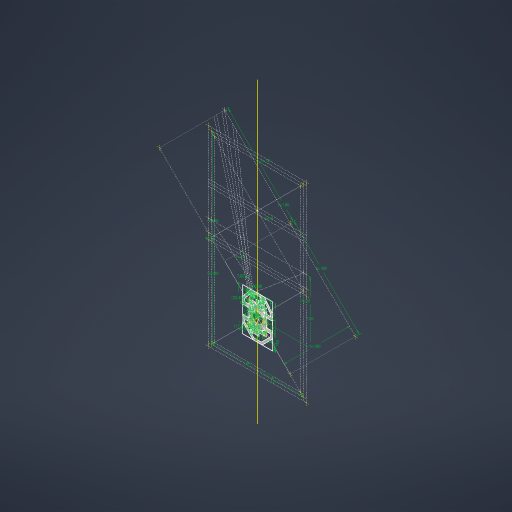
# Autodesk Inventor part: chassis
Saved by Autodesk Inventor 2023.5 (Build 275446000, 446)
## iProperties
Created: 2025-01-19
Part Number: chassis
Material: 一般
Document SubType Name: Modeling
Designer: IshiiLabHonda
Density: 1 g/cm^3
Appearance: 既定
Author: IshiiLabHonda
Autodesk Inventor part; units mm, degrees
ref_plane "YZ Plane" through (0, 0, 0) normal (1, 0, 0) x (0, 1, 0)
ref_plane "XZ Plane" through (0, 0, 0) normal (0, 1, 0) x (-1, 0, 0)
ref_plane "XY Plane" through (0, 0, 0) normal (0, 0, 1) x (1, 0, 0)
sketch "スケッチ1" plane through (0, 0, 0) normal (0, 0, 1) x (1, 0, 0)
  line L0 (-90, 90) -> (90, 90) construction
  line L1 (90, 90) -> (90, -90) construction
  line L2 (90, -90) -> (-90, -90) construction
  line L3 (-90, -90) -> (-90, 90) construction
  line L4 (-90, 90) -> (-90, 270) construction
  line L5 (-90, 270) -> (90, 270) construction
  line L6 (90, 270) -> (90, 90) construction
  line L7 (-90, 90) -> (90, -90) construction
  line L8 (90, 90) -> (-90, -90) construction
  line L9 (0, 0) -> (0, 10) construction
  line L10 (0, 0) -> (10, 0) construction
  line L11 (-90, 270) -> (90, 90) construction
  line L12 (-90, 90) -> (90, 270) construction
  line L13 (-96, 276) -> (96, 276) construction
  line L14 (96, 276) -> (96, -96) construction
  line L15 (96, -96) -> (-96, -96) construction
  line L16 (-96, -96) -> (-96, 276) construction
  line L17 (-84, 264) -> (84, 264) construction
  line L18 (84, 264) -> (84, -84) construction
  line L19 (84, -84) -> (-84, -84) construction
  line L20 (-84, -84) -> (-84, 264) construction
  line L21 (-96, 96) -> (96, 96) construction
  line L22 (-96, 84) -> (96, 84) construction
  line L23 (-63.6396, 63.6396) -> (63.6396, 190.9188) construction
  line L24 (63.6396, 190.9188) -> (190.9188, 63.6396) construction
  line L25 (190.9188, 63.6396) -> (63.6396, -63.6396) construction
  line L26 (63.6396, -63.6396) -> (-63.6396, 63.6396) construction
  line L27 (-190.9188, 190.9188) -> (-63.6396, 318.1981) construction
  line L28 (-63.6396, 318.1981) -> (63.6396, 190.9188) construction
  line L29 (-63.6396, 63.6396) -> (-190.9188, 190.9188) construction
  line L30 (-96, 120) -> (96, 120) construction
  line L31 (-96, 186) -> (96, 186) construction
  line L32 (-96, 174) -> (96, 174) construction
  line L33 (-96, 180) -> (96, 180) construction
  point P0 (-63.6396, 318.1981)
  point P1 (-90, 120)
  point P2 (90, 120)
  point P3 (0, 180)
  dimension "d8" = 10
  dimension "d9" = 10
  dimension "d10" = 12
  dimension "d11" = 12
  dimension "d12" = 12
  dimension "d13" = 12
  dimension "d14" = 180
  dimension "d15" = 180
  dimension "d16" = 180
  dimension "d17" = 12
  dimension "d34" = 180
  dimension "d35" = 180
  dimension "d36" = 180
  dimension "d37" = 120
  dimension "d85" = 12
  constraints: 68 end point, 16 parallel, 16 point on line, 9 perpendicular, 4 midpoint, 3 coincident, 1 horizontal, 7 other
  measures "d8" distance of L9.start L9.end
  measures "d9" distance of L9.start L10.end
  measures "d10" distance between parallel lines of L15 L19
  measures "d11" distance between parallel lines of L16 L20
  measures "d12" distance between parallel lines of L14 L18
  measures "d13" distance between parallel lines of L17 L13
  measures "d14" distance of L1.end L2.end
  measures "d15" distance of L2.end L0.start
  measures "d16" distance between parallel lines of L0 L5
  measures "d17" distance between parallel lines of L22 L21
  measures "d34" distance between parallel lines of L26 L24
  measures "d35" distance of L23.end L24.end
  measures "d36" distance between parallel lines of L23 L27
  measures "d37" distance between parallel lines of L10 L30
  measures "d85" distance between parallel lines of L32 L31
sketch "スケッチ2" plane through (0, 0, 0) normal (0, 0, 1) x (1, 0, 0)
  line L0 (63.6396, 190.9188) -> (190.9188, 63.6396) construction
  line L1 (-63.6396, 318.1981) -> (63.6396, 190.9188) construction
  line L2 (-84, 264) -> (84, 264) construction
  line L3 (-90, 270) -> (90, 270) construction
  line L4 (90, 270) -> (90, 90) construction
  line L5 (-96, 276) -> (96, 276) construction
  line L6 (-90, 90) -> (90, 270) construction
  line L7 (-90, 270) -> (90, 90) construction
  line L8 (-63.6396, 63.6396) -> (63.6396, 190.9188) construction
  line L9 (-96, 120) -> (96, 120) construction
  line L10 (-90, 90) -> (90, 90) construction
  line L11 (-96, 96) -> (96, 96) construction
  line L12 (-96, 84) -> (96, 84) construction
  line L13 (90, -90) -> (-90, -90) construction
  line L14 (0, 0) -> (0, 10) construction
  line L15 (0, 0) -> (10, 0) construction
  line L16 (190.9188, 63.6396) -> (63.6396, -63.6396) construction
  line L17 (63.6396, -63.6396) -> (-63.6396, 63.6396) construction
  line L18 (84, -84) -> (-84, -84) construction
  line L19 (96, -96) -> (-96, -96) construction
  line L20 (-90, 90) -> (-90, 270) construction
  line L21 (-63.6396, 63.6396) -> (-190.9188, 190.9188) construction
  line L22 (-190.9188, 190.9188) -> (-63.6396, 318.1981) construction
  line L23 (96, 276) -> (96, -96) construction
  line L24 (-96, -96) -> (-96, 276) construction
  line L25 (84, 264) -> (84, -84) construction
  line L26 (-84, -84) -> (-84, 264) construction
  line L27 (90, 90) -> (90, -90) construction
  line L28 (-90, 90) -> (90, -90) construction
  line L29 (90, 90) -> (-90, -90) construction
  line L30 (-90, -90) -> (-90, 90) construction
  circle A0 centre (0, 0) radius 16.5 construction
  circle A1 centre (0, 0) radius 10 construction
  line L31 (20, 11.5) -> (28.75, 11.5) construction
  line L32 (28.75, 11.5) -> (28.75, -11.5) construction
  line L33 (28.75, -11.5) -> (20, -11.5) construction
  line L34 (20, -11.5) -> (20, 11.5) construction
  line L35 (20, 11.5) -> (18, 11.5) construction
  line L36 (18, 11.5) -> (18, -11.5) construction
  line L37 (18, -11.5) -> (20, -11.5) construction
  line L38 (18, 1.5) -> (17, 1.5) construction
  line L39 (17, -1.5) -> (18, -1.5) construction
  line L40 (-17, 24) -> (17, 24) construction
  line L41 (17, 24) -> (17, -24) construction
  line L42 (17, -24) -> (-17, -24) construction
  line L43 (-17, -24) -> (-17, 24) construction
  line L44 (-20, 11.5) -> (-28.75, 11.5) construction
  line L45 (-28.75, 11.5) -> (-28.75, -11.5) construction
  line L46 (-28.75, -11.5) -> (-20, -11.5) construction
  line L47 (-20, -11.5) -> (-20, 11.5) construction
  line L48 (-20, 11.5) -> (-18, 11.5) construction
  line L49 (-18, 11.5) -> (-18, -11.5) construction
  line L50 (-18, -11.5) -> (-20, -11.5) construction
  line L51 (-18, 1.5) -> (-17, 1.5) construction
  line L52 (-17, -1.5) -> (-18, -1.5) construction
  line L53 (-14.5, 24) -> (-14.5, -24) construction
  line L54 (14.5, 24) -> (14.5, -24) construction
  line L55 (-10.5, 24) -> (-10.5, 19) construction
  line L56 (-10.5, 19) -> (-14.5, 19) construction
  line L57 (-14.5, 24) -> (-10.5, 19) construction
  line L58 (-10.5, 24) -> (-14.5, 19) construction
  circle A2 centre (-12.5, 21.5) radius 1 construction
  line L59 (10.5, 24) -> (10.5, 19) construction
  line L60 (10.5, 19) -> (14.5, 19) construction
  line L61 (10.5, 24) -> (14.5, 19) construction
  line L62 (10.5, 19) -> (14.5, 24) construction
  circle A3 centre (12.5, 21.5) radius 1 construction
  line L63 (-14.5, -19) -> (-10.5, -19) construction
  line L64 (-10.5, -19) -> (-10.5, -24) construction
  line L65 (10.5, -24) -> (10.5, -19) construction
  line L66 (10.5, -19) -> (14.5, -19) construction
  line L67 (-14.5, -19) -> (-10.5, -24) construction
  line L68 (-10.5, -19) -> (-14.5, -24) construction
  circle A4 centre (-12.5, -21.5) radius 1 construction
  line L69 (10.5, -19) -> (14.5, -24) construction
  line L70 (14.5, -19) -> (10.5, -24) construction
  circle A5 centre (12.5, -21.5) radius 1 construction
  point P0 (90, 120)
  point P1 (-90, 120)
  point P2 (-63.6396, 318.1981)
  point P3 (-12.5, -21.5)
  point P4 (-12.5, 21.5)
  dimension "d38" = 33
  dimension "d39" = 20
  dimension "d40" = 8.75
  dimension "d41" = 2
  dimension "d42" = 23
  dimension "d44" = 3
  dimension "d45" = 1
  dimension "d48" = 2.5
  dimension "d49" = 24
  dimension "d50" = 24
  dimension "d51" = 2
  dimension "d52" = 5
  dimension "d53" = 4
  dimension "d54" = 2
  dimension "d55" = 4
  dimension "d56" = 5
  dimension "d57" = 2
  dimension "d58" = 4
  dimension "d59" = 5
  dimension "d60" = 2
  dimension "d61" = 5
  dimension "d62" = 4
  dimension "d63" = 57.5
  dimension "d71" = 43
  dimension "d154" = 29
  constraints: 80 end point, 18 point on line, 12 parallel, 10 symmetric about line, 6 centre point, 6 midpoint, 6 perpendicular, 2 coincident, 2 collinear, 5 other
  measures "d38" diameter of A0
  measures "d39" diameter of A1
  measures "d40" distance between parallel lines of L34 L32
  measures "d41" distance between parallel lines of L36 L34
  measures "d42" distance between parallel lines of L33 L31
  measures "d44" distance between parallel lines of L39 L38
  measures "d45" distance between parallel lines of L41 L36
  measures "d48" distance between parallel lines of L43 L53
  measures "d49" distance between parallel lines of L42 L15
  measures "d50" distance between parallel lines of L15 L40
  measures "d51" diameter of A2
  measures "d52" distance of L55.start L55.end
  measures "d53" distance of L55.end L56.end
  measures "d54" diameter of A3
  measures "d55" distance of L59.end L60.end
  measures "d56" distance of L59.start L59.end
  measures "d57" diameter of A4
  measures "d58" distance of L63.start L63.end
  measures "d59" distance of L63.end L64.end
  measures "d60" diameter of A5
  measures "d61" distance of L65.start L65.end
  measures "d62" distance of L65.end L66.end
  measures "d63" distance between parallel lines of L32 L45
  measures "d71" distance of point (-12.5, -21.5) point (-12.5, 21.5)
  measures "d154" distance between parallel lines of L54 L53
sketch "スケッチ3" plane through (0, 0, 0) normal (0, 0, 1) x (1, 0, 0)
  line L0 (63.6396, 190.9188) -> (190.9188, 63.6396) construction
  line L1 (-63.6396, 318.1981) -> (63.6396, 190.9188) construction
  line L2 (-84, 264) -> (84, 264) construction
  line L3 (-90, 270) -> (90, 270) construction
  line L4 (90, 270) -> (90, 90) construction
  line L5 (-96, 276) -> (96, 276) construction
  line L6 (-90, 90) -> (90, 270) construction
  line L7 (-90, 270) -> (90, 90) construction
  line L8 (-63.6396, 63.6396) -> (63.6396, 190.9188) construction
  line L9 (-96, 120) -> (96, 120) construction
  line L10 (-90, 90) -> (90, 90) construction
  line L11 (-96, 96) -> (96, 96) construction
  line L12 (-96, 84) -> (96, 84) construction
  line L13 (90, -90) -> (-90, -90) construction
  line L14 (0, 0) -> (0, 10) construction
  line L15 (0, 0) -> (10, 0) construction
  line L16 (190.9188, 63.6396) -> (63.6396, -63.6396) construction
  line L17 (63.6396, -63.6396) -> (-63.6396, 63.6396) construction
  line L18 (84, -84) -> (-84, -84) construction
  line L19 (96, -96) -> (-96, -96) construction
  line L20 (-90, 90) -> (-90, 270) construction
  line L21 (-63.6396, 63.6396) -> (-190.9188, 190.9188) construction
  line L22 (-190.9188, 190.9188) -> (-63.6396, 318.1981) construction
  line L23 (96, 276) -> (96, -96) construction
  line L24 (-96, -96) -> (-96, 276) construction
  line L25 (84, 264) -> (84, -84) construction
  line L26 (-84, -84) -> (-84, 264) construction
  line L27 (90, 90) -> (90, -90) construction
  line L28 (-90, 90) -> (90, -90) construction
  line L29 (90, 90) -> (-90, -90) construction
  line L30 (-90, -90) -> (-90, 90) construction
  line L31 (-18, 1.5) -> (-17, 1.5) construction
  line L32 (-17, -1.5) -> (-18, -1.5) construction
  line L33 (-20, 11.5) -> (-18, 11.5) construction
  line L34 (-28.75, 11.5) -> (-28.75, -11.5) construction
  line L35 (63.6396, -63.6396) -> (-63.6396, 63.6396) construction
  line L36 (84, -84) -> (-84, -84) construction
  line L37 (-90, -90) -> (-90, 90) construction
  line L38 (96, -96) -> (-96, -96) construction
  line L39 (-90, 90) -> (90, 90) construction
  line L40 (90, -90) -> (-90, -90) construction
  line L41 (90, 90) -> (-90, -90) construction
  line L42 (-90, 90) -> (90, -90) construction
  line L43 (90, 90) -> (90, -90) construction
  line L44 (-28.75, -11.5) -> (-20, -11.5) construction
  line L45 (-20, 11.5) -> (-28.75, 11.5) construction
  line L46 (-18, 11.5) -> (-18, -11.5) construction
  line L47 (-18, -11.5) -> (-20, -11.5) construction
  line L48 (0, 0) -> (0, 10) construction
  line L49 (0, 0) -> (10, 0) construction
  circle A0 centre (0, 0) radius 16.5 construction
  circle A1 centre (0, 0) radius 10 projected
  line L50 (-14.5, 24) -> (-14.5, -24) construction
  line L51 (-17, 24) -> (17, 24) construction
  line L52 (-17, -24) -> (-17, 24) construction
  line L53 (17, -24) -> (-17, -24) construction
  line L54 (-14.5, -19) -> (-10.5, -19) construction
  circle A2 centre (-12.5, -21.5) radius 1 projected
  line L55 (-10.5, -19) -> (-14.5, -24) construction
  line L56 (-14.5, -19) -> (-10.5, -24) construction
  line L57 (-63.6396, 318.1981) -> (63.6396, 190.9188) construction
  line L58 (-84, 264) -> (84, 264) construction
  line L59 (-90, 270) -> (90, 270) construction
  line L60 (90, 270) -> (90, 90) construction
  line L61 (-96, 276) -> (96, 276) construction
  line L62 (-90, 90) -> (90, 270) construction
  line L63 (-90, 270) -> (90, 90) construction
  line L64 (-63.6396, 63.6396) -> (63.6396, 190.9188) construction
  line L65 (-96, 120) -> (96, 120) construction
  line L66 (-96, 96) -> (96, 96) construction
  line L67 (-96, 84) -> (96, 84) construction
  line L68 (84, 264) -> (84, -84) construction
  line L69 (96, 276) -> (96, -96) construction
  line L70 (-96, -96) -> (-96, 276) construction
  line L71 (-84, -84) -> (-84, 264) construction
  line L72 (-63.6396, 63.6396) -> (-190.9188, 190.9188) construction
  line L73 (-90, 90) -> (-90, 270) construction
  line L74 (-190.9188, 190.9188) -> (-63.6396, 318.1981) construction
  line L75 (-20, -11.5) -> (-20, 11.5) construction
  line L76 (10.5, -19) -> (14.5, -19) construction
  line L77 (10.5, -24) -> (10.5, -19) construction
  circle A3 centre (12.5, -21.5) radius 1 projected
  line L78 (10.5, -19) -> (14.5, -24) construction
  line L79 (14.5, -19) -> (10.5, -24) construction
  line L80 (-10.5, -19) -> (-10.5, -24) construction
  line L81 (63.6396, 190.9188) -> (190.9188, 63.6396) construction
  line L82 (190.9188, 63.6396) -> (63.6396, -63.6396) construction
  line L83 (20, 11.5) -> (28.75, 11.5) construction
  line L84 (28.75, 11.5) -> (28.75, -11.5) construction
  line L85 (17, -1.5) -> (18, -1.5) construction
  line L86 (18, -11.5) -> (20, -11.5) construction
  line L87 (28.75, -11.5) -> (20, -11.5) construction
  line L88 (14.5, 24) -> (14.5, -24) construction
  line L89 (17, 24) -> (17, -24) construction
  line L90 (18, 11.5) -> (18, -11.5) construction
  line L91 (20, -11.5) -> (20, 11.5) construction
  line L92 (20, 11.5) -> (18, 11.5) construction
  line L93 (18, 1.5) -> (17, 1.5) construction
  line L94 (-10.5, 24) -> (-10.5, 19) construction
  line L95 (10.5, 19) -> (14.5, 19) construction
  circle A4 centre (12.5, 21.5) radius 1 projected
  line L96 (10.5, 24) -> (14.5, 19) construction
  line L97 (10.5, 19) -> (14.5, 24) construction
  line L98 (10.5, 24) -> (10.5, 19) construction
  line L99 (-10.5, 19) -> (-14.5, 19) construction
  circle A5 centre (-12.5, 21.5) radius 1 projected
  line L100 (-14.5, 24) -> (-10.5, 19) construction
  line L101 (-10.5, 24) -> (-14.5, 19) construction
  line L102 (29.25, 41.5) -> (29.25, -41.5)
  line L103 (-29.25, -41.5) -> (-29.25, 41.5)
  line L104 (-29.25, 8.5) -> (-17, 8.5)
  line L105 (-17, 8.5) -> (-17, -8.5)
  line L106 (-17, -8.5) -> (-29.25, -8.5)
  line L107 (29.25, 8.5) -> (17, 8.5)
  line L108 (17, 8.5) -> (17, -8.5)
  line L109 (17, -8.5) -> (29.25, -8.5)
  line L110 (10.0101, 40.6505) -> (14.9894, 36.4724) construction
  line L111 (10.4899, 31.11) -> (12.788, 29.1817) construction
  line L112 (12.788, 29.1817) -> (17.2875, 34.544) construction
  line L113 (10.5581, 32.3582) -> (9.9419, 39.4023) construction
  line L114 (17.2875, 34.544) -> (14.9894, 36.4724) construction
  line L115 (10.4899, 31.11) -> (5.5106, 35.2882) construction
  line L116 (10.5581, 32.3582) -> (6.7279, 35.5721) construction
  line L117 (6.7279, 35.5721) -> (9.9419, 39.4023) construction
  line L118 (5.5106, 35.2882) -> (10.0101, 40.6505) construction
  line L119 (10.0101, 40.6505) -> (10.4899, 31.11) construction
  line L120 (13.7721, 36.1884) -> (10.5581, 32.3582) construction
  line L121 (6.7279, 35.5721) -> (13.7721, 36.1884) construction
  line L122 (5.5106, 35.2882) -> (14.9894, 36.4724) construction
  line L123 (14.9894, 36.4724) -> (10.4899, 31.11) construction
  line L124 (9.9419, 39.4023) -> (13.7721, 36.1884) construction
  line L125 (-7.6191, 6.1457) -> (-8.4873, 11.0698) construction
  line L126 (-2.7087, 12.8503) -> (-1.1893, 4.2332) construction
  line L127 (-3.5633, 11.938) -> (-2.695, 7.014) construction
  line L128 (-7.6191, 6.1457) -> (-3.5633, 11.938) construction
  line L129 (-8.4873, 11.0698) -> (-2.695, 7.014) construction
  line L130 (-9.1099, 11.7216) -> (-2.7087, 12.8503) construction
  line L131 (-1.1893, 4.2332) -> (-7.5905, 3.1045) construction
  line L132 (-63.6396, 318.1981) -> (-5.5912, 9.0419) construction
  line L133 (10.25, 35.8803) -> (-90, 120) construction
  line L134 (-5.5912, 9.0419) -> (-79.4589, 302.3788) construction
  line L135 (-5.5912, 9.0419) -> (-41.5175, 296.076) construction
  line L136 (-9.9419, 39.4023) -> (-6.7279, 35.5721) construction
  line L137 (-10.0101, 40.6505) -> (-5.5106, 35.2882) construction
  line L138 (-14.9894, 36.4724) -> (-10.0101, 40.6505) construction
  line L139 (-5.5106, 35.2882) -> (-14.9894, 36.4724) construction
  line L140 (-13.7721, 36.1884) -> (-6.7279, 35.5721) construction
  line L141 (-13.7721, 36.1884) -> (-9.9419, 39.4023) construction
  line L142 (-14.9894, 36.4724) -> (-17.2875, 34.544) construction
  line L143 (-6.7279, 35.5721) -> (-10.5581, 32.3582) construction
  line L144 (-9.9419, 39.4023) -> (-10.5581, 32.3582) construction
  line L145 (-10.5581, 32.3582) -> (-13.7721, 36.1884) construction
  line L146 (-10.0101, 40.6505) -> (-10.4899, 31.11) construction
  line L147 (-5.5106, 35.2882) -> (-10.4899, 31.11) construction
  line L148 (-10.4899, 31.11) -> (-14.9894, 36.4724) construction
  line L149 (-17.2875, 34.544) -> (-12.788, 29.1817) construction
  line L150 (-12.788, 29.1817) -> (-10.4899, 31.11) construction
  line L151 (-10.25, 35.8803) -> (90, 120) construction
  circle A6 centre (-7.0361, 32.05) radius 0.625 construction
  circle A7 centre (-7.0361, 32.05) radius 0.8
  circle A8 centre (-7.0361, 32.05) radius 1.5 construction
  circle A9 centre (-16.0715, 34.6506) radius 0.625 construction
  circle A10 centre (-16.0715, 34.6506) radius 0.8
  circle A11 centre (-16.0715, 34.6506) radius 1.5 construction
  line L152 (-2.695, 7.014) -> (-7.6191, 6.1457) construction
  line L153 (-7.9812, 5.3203) -> (-1.58, 6.449) construction
  line L154 (-8.0532, 8.6078) -> (-3.1291, 9.476) construction
  line L155 (-4.6361, 3.6254) -> (-5.157, 6.5799) construction
  line L156 (-8.4873, 11.0698) -> (-3.5633, 11.938) construction
  circle A12 centre (7.0361, 32.05) radius 0.625 construction
  circle A13 centre (7.0361, 32.05) radius 0.8
  circle A14 centre (7.0361, 32.05) radius 1.5 construction
  circle A15 centre (16.0715, 34.6506) radius 1.5 construction
  circle A16 centre (16.0715, 34.6506) radius 0.8
  circle A17 centre (16.0715, 34.6506) radius 0.625 construction
  line L157 (-29.25, -41.5) -> (29.25, -41.5)
  line L158 (-29.25, 41.5) -> (29.25, 41.5)
  line L159 (-10.25, 35.8803) -> (-7.0361, 32.05) construction
  line L160 (-29.25, 20.8653) -> (-13.3068, 41.5)
  line L161 (-29.25, -21.1569) -> (-8.9069, -41.5)
  line L162 (29.25, 20.8653) -> (13.3068, 41.5)
  line L163 (29.25, -21.1569) -> (8.9069, -41.5)
  line L164 (25.25, 19.5) -> (25.25, 14.5)
  line L165 (25.25, 14.5) -> (17, 14.5)
  line L166 (-17, 14.5) -> (-25.25, 14.5)
  line L167 (-25.25, 14.5) -> (-25.25, 19.5)
  line L168 (2.7087, 12.8503) -> (1.1893, 4.2332) construction
  line L169 (3.5633, 11.938) -> (2.695, 7.014) construction
  line L170 (8.4873, 11.0698) -> (2.695, 7.014) construction
  line L171 (7.6191, 6.1457) -> (3.5633, 11.938) construction
  line L172 (9.1099, 11.7216) -> (2.7087, 12.8503) construction
  line L173 (7.6191, 6.1457) -> (8.4873, 11.0698) construction
  line L174 (1.1893, 4.2332) -> (7.5905, 3.1045) construction
  line L175 (7.5905, 3.1045) -> (9.1099, 11.7216) construction
  line L176 (2.695, 7.014) -> (7.6191, 6.1457) construction
  line L177 (7.9812, 5.3203) -> (1.58, 6.449) construction
  line L178 (8.4873, 11.0698) -> (3.5633, 11.938) construction
  line L179 (13.5, 30) -> (13.5, 24)
  line L180 (13.5, 24) -> (17, 24)
  line L181 (17, 24) -> (17, 14.5)
  line L182 (-13.5, 24) -> (-17, 24)
  line L183 (-17, 24) -> (-17, 14.5)
  line L184 (-17, -14.5) -> (-25.25, -14.5)
  line L185 (-25.25, -14.5) -> (-25.25, -19.5)
  line L186 (-25.25, -19.5) -> (-7.25, -37.5)
  line L187 (-7.25, -37.5) -> (7.25, -37.5)
  line L188 (7.25, -37.5) -> (25.25, -19.5)
  line L189 (25.25, -19.5) -> (25.25, -14.5)
  line L190 (25.25, -14.5) -> (17, -14.5)
  line L191 (17, -14.5) -> (17, -24)
  line L192 (17, -24) -> (13.5, -24)
  line L193 (-13.5, -30) -> (-13.5, -24)
  line L194 (-13.5, -24) -> (-17, -24)
  line L195 (-17, -24) -> (-17, -14.5)
  line L196 (-9.1099, 11.7216) -> (-7.5905, 3.1045) construction
  line L197 (-9.4721, 10.8961) -> (-8.6039, 5.9721) construction
  line L198 (-14.3961, 10.0279) -> (-8.6039, 5.9721) construction
  line L199 (-13.5279, 5.1039) -> (-9.4721, 10.8961) construction
  line L200 (-15.5112, 10.5929) -> (-9.1099, 11.7216) construction
  line L201 (-13.5279, 5.1039) -> (-14.3961, 10.0279) construction
  line L202 (-7.5905, 3.1045) -> (-13.9918, 1.9758) construction
  line L203 (-8.6039, 5.9721) -> (-13.5279, 5.1039) construction
  line L204 (-13.962, 7.5659) -> (-9.038, 8.4341) construction
  line L205 (-10.5449, 2.5836) -> (-11.0659, 5.538) construction
  line L206 (-14.3961, 10.0279) -> (-9.4721, 10.8961) construction
  line L207 (9.1099, 11.7216) -> (7.5905, 3.1045) construction
  line L208 (9.4721, 10.8961) -> (8.6039, 5.9721) construction
  line L209 (14.3961, 10.0279) -> (8.6039, 5.9721) construction
  line L210 (13.5279, 5.1039) -> (9.4721, 10.8961) construction
  line L211 (13.5279, 5.1039) -> (14.3961, 10.0279) construction
  line L212 (7.5905, 3.1045) -> (13.9918, 1.9758) construction
  line L213 (13.9918, 1.9758) -> (15.5112, 10.5929) construction
  line L214 (14.3961, 10.0279) -> (9.4721, 10.8961) construction
  line L215 (13.962, 7.5659) -> (9.038, 8.4341) construction
  line L216 (8.6039, 5.9721) -> (13.5279, 5.1039) construction
  line L217 (10.5449, 2.5836) -> (11.0659, 5.538) construction
  line L218 (15.5112, 10.5929) -> (9.1099, 11.7216) construction
  line L219 (-25.25, 19.5) -> (-11.3425, 37.5)
  line L220 (-11.3425, 37.5) -> (11.3425, 37.5)
  line L221 (11.3425, 37.5) -> (25.25, 19.5)
  circle A18 centre (0, 0) radius 4.25 construction
  line L222 (-11.5, 8) -> (-68.7791, 313.0586) construction
  line L223 (-11.5, 8) -> (-84.3887, 297.449) construction
  line L224 (-11.5, 8) -> (-48.4208, 302.9793) construction
  line L225 (-15.5112, 10.5929) -> (-13.9918, 1.9758) construction
  line L226 (-14.3825, 4.1916) -> (-7.9812, 5.3203) construction
  circle A19 centre (-10.5, -27) radius 1
  circle A20 centre (10.5, 27) radius 1
  circle A21 centre (10.5, 27) radius 2
  circle A22 centre (-10.5, -27) radius 2
  circle A23 centre (0, -27) radius 1
  circle A24 centre (0, -27) radius 2
  circle A25 centre (0, 27) radius 1
  circle A26 centre (0, 27) radius 2
  line L227 (0, 27) -> (10.5, 27) construction
  line L228 (-10.5, -27) -> (0, -27) construction
  line L229 (13.5, 30) -> (-3, 30)
  line L230 (-3, 30) -> (-3, 24)
  line L231 (-13.5, 24) -> (-3, 24)
  line L232 (-13.5, -30) -> (3, -30)
  line L233 (3, -30) -> (3, -24)
  line L234 (3, -24) -> (13.5, -24)
  line L235 (-16.1606, 31.2641) -> (-6.1594, 29.9135)
  line L236 (-6.1594, 29.9135) -> (-5.0634, 31.332)
  line L237 (-5.0634, 31.332) -> (-4.8147, 37.5)
  line L238 (16.1606, 31.2641) -> (6.1594, 29.9135)
  line L239 (6.1594, 29.9135) -> (5.0634, 31.332)
  line L240 (5.0634, 31.332) -> (4.8147, 37.5)
  line L241 (-10.5, -27) -> (-14.125, -30.625) construction
  line L242 (-15.5392, -29.2108) -> (-13.5, -24)
  line L243 (-12.7108, -32.0392) -> (-7.5, -30)
  line L244 (10.5, 27) -> (13.5, 30) construction
  line L245 (16.1606, 31.2641) -> (10.0926, 30)
  line L246 (-10.5, -19) -> (-10.5, -20.4081)
  line L247 (-10.5, -20.4081) -> (-7.5, -21.5)
  line L248 (-7.5, -21.5) -> (7.5, -21.5)
  line L249 (7.5, -21.5) -> (10.5, -20.4081)
  line L250 (10.5, -20.4081) -> (10.5, -19)
  line L251 (10.5, -19) -> (-10.5, -19)
  line L252 (-10.5, 19) -> (-10.5, 20.4081)
  line L253 (-10.5, 20.4081) -> (-7.5, 21.5)
  line L254 (-7.5, 21.5) -> (7.5, 21.5)
  line L255 (7.5, 21.5) -> (10.5, 20.4081)
  line L256 (10.5, 20.4081) -> (10.5, 19)
  line L257 (10.5, 19) -> (-10.5, 19)
  line L258 (-5.3602, -19) -> (-14.5, -13.3971)
  line L259 (-14.5, -13.3971) -> (-14.5, -15.3971)
  line L260 (0, 0) -> (-9.9301, -16.1985) construction
  line L261 (5.3602, -19) -> (14.5, -13.3971)
  line L262 (14.5, -13.3971) -> (14.5, -15.3971)
  line L263 (-5.3602, 19) -> (-14.5, 13.3971)
  line L264 (-14.5, 13.3971) -> (-14.5, 15.3971)
  line L265 (14.5, 13.3971) -> (14.5, 15.3971)
  line L266 (5.3602, 19) -> (14.5, 13.3971)
  line L267 (-14.5, -15.3971) -> (-10.5, -20.4081)
  line L268 (10.5, -20.4081) -> (14.5, -15.3971)
  line L269 (-14.5, 15.3971) -> (-10.5, 20.4081)
  line L270 (14.5, 15.3971) -> (10.5, 20.4081)
  line L271 (-5.3602, -19) -> (-9.4462, -17.5128)
  line L272 (-9.4462, -17.5128) -> (-14.5, -13.3971)
  line L273 (-10.5, -20.4081) -> (-9.4462, -17.5128) construction
  line L274 (5.3602, -19) -> (9.4462, -17.5128)
  line L275 (9.4462, -17.5128) -> (14.5, -13.3971)
  line L276 (-5.3602, 19) -> (-9.4462, 17.5128)
  line L277 (-9.4462, 17.5128) -> (-14.5, 13.3971)
  line L278 (9.4462, 17.5128) -> (14.5, 13.3971)
  line L279 (5.3602, 19) -> (9.4462, 17.5128)
  point P0 (29.25, -8.5)
  point P1 (29.25, 8.5)
  point P2 (29.25, -21.1569)
  point P3 (8.9069, -41.5)
  point P4 (13.3068, 41.5)
  point P5 (29.25, 20.8653)
  point P6 (-4.8676, -26)
  point P7 (11.5, 8)
  point P8 (11.5, 8)
  point P9 (-5.5912, 9.0419)
  point P10 (-5.5912, 9.0419)
  point P11 (-12.75, -30)
  point P12 (-13.5, -29.25)
  point P13 (12.75, 30)
  point P14 (13.5, 29.25)
  point P15 (-16.4572, 33.9497)
  point P16 (-15.3706, 35.0362)
  point P17 (15.3706, 35.0362)
  point P18 (16.4572, 33.9497)
  point P19 (6.2577, 30)
  point P20 (6.8, 30)
  point P21 (16.1606, 31.2641)
  point P22 (13.6038, 24)
  point P23 (-12.7108, -32.0392)
  point P24 (6.0926, 30)
  dimension "d78" = 17
  dimension "d80" = 0.5
  dimension "d81" = 58.5
  dimension "d82" = 57.5
  dimension "d84" = 0
  dimension "d119" = 5
  dimension "d123" = 5
  dimension "d124" = 5
  dimension "d125" = 6.5
  dimension "d126" = 7
  dimension "d127" = 3
  dimension "d128" = 7
  dimension "d130" = 5
  dimension "d131" = 5
  dimension "d132" = 6.5
  dimension "d133" = 7
  dimension "d134" = 3
  dimension "d135" = 100
  dimension "d141" = 1.25
  dimension "d142" = 1.6
  dimension "d143" = 3
  dimension "d144" = 1.25
  dimension "d145" = 1.6
  dimension "d146" = 3
  dimension "d156" = 3
  dimension "d157" = 6.5
  dimension "d173" = 5
  dimension "d187" = 83
  dimension "d194" = 41.5
  dimension "d198" = 45
  dimension "d205" = 0
  dimension "d206" = 4
  dimension "d207" = 4
  dimension "d208" = 4
  dimension "d209" = 4
  dimension "d210" = 6
  dimension "d211" = 6
  dimension "d263" = 5
  dimension "d264" = 3
  dimension "d267" = 5
  dimension "d269" = 32.4581
  dimension "d273" = 41.5
  dimension "d274" = 17.5
  dimension "d316" = 8.5
  dimension "d317" = 7
  dimension "d319" = 1
  dimension "d320" = 1
  dimension "d324" = 1
  dimension "d327" = 3
  dimension "d328" = 8
  dimension "d329" = 10
  dimension "d330" = 2
  dimension "d331" = 2
  dimension "d334" = 4
  dimension "d335" = 4
  dimension "d338" = 2
  dimension "d339" = 4
  dimension "d340" = 2
  dimension "d341" = 4
  dimension "d342" = 3
  dimension "d343" = 3
  dimension "d344" = 10.5
  dimension "d345" = 10.5
  dimension "d346" = 1
  constraints: 356 end point, 59 horizontal alignment, 41 parallel, 41 point on line, 38 perpendicular, 24 midpoint, 21 centre point, 14 vertical alignment, 13 coincident, 6 equal radius, 6 horizontal, 2 symmetric about line, 1 collinear, 1 tangent, 1 vertical, 22 other
  measures "d78" distance between parallel lines of L106 L104
  measures "d80" distance between parallel lines of L103 L34
  measures "d81" distance between parallel lines of L102 L103
  measures "d82" distance between parallel lines of L84 L34
  measures "d84" distance between parallel lines of L105 L52
  measures "d119" distance between parallel lines of L125 L127
  measures "d123" distance between parallel lines of L120 L117
  measures "d124" distance of L124.end L113.start
  measures "d125" distance between parallel lines of L123 L118
  measures "d126" distance between parallel lines of L110 L115
  measures "d127" distance between parallel lines of L112 L123
  measures "d128" angle of L134 L135
  measures "d130" distance between parallel lines of L145 L136
  measures "d131" distance of L143.end L140.start
  measures "d132" distance between parallel lines of L148 L137
  measures "d133" distance between parallel lines of L147 L138
  measures "d134" distance between parallel lines of L149 L148
  measures "d135" angle of L133 L151
  measures "d141" diameter of A6
  measures "d142" diameter of A7
  measures "d143" diameter of A8
  measures "d144" diameter of A9
  measures "d145" diameter of A10
  measures "d146" diameter of A11
  measures "d156" distance between parallel lines of L131 L152
  measures "d157" distance between parallel lines of L153 L130
  measures "d173" distance of L128.start L129.start
  measures "d187" distance between parallel lines of L157 L158
  measures "d194" distance of the line from the sketch origin of L157
  measures "d198" angle of L103 L161
  measures "d205" distance between parallel lines of L183 L52
  measures "d206" distance between parallel lines of L103 L167
  measures "d207" distance between parallel lines of L157 L187
  measures "d208" distance between parallel lines of L161 L186
  measures "d209" distance between parallel lines of L103 L185
  measures "d210" distance between parallel lines of L184 L106
  measures "d211" distance between parallel lines of L104 L166
  measures "d263" distance between parallel lines of L201 L197
  measures "d264" distance between parallel lines of L202 L203
  measures "d267" distance of L199.start L198.start
  measures "d269" distance from line of L158 point (-5.591, 9.042)
  measures "d273" distance of the line from the sketch origin of L158
  measures "d274" distance between parallel lines of L157 L194
  measures "d316" diameter of A18
  measures "d317" angle of L223 L224
  measures "d319" distance between parallel lines of L127 L126
  measures "d320" distance between parallel lines of L197 L125
  measures "d324" distance between parallel lines of L225 L201
  measures "d327" distance from line of L50 L222.start
  measures "d329" angle to the sketch x axis of L202
  measures "d330" diameter of A19
  measures "d331" diameter of A20
  measures "d334" diameter of A21
  measures "d335" diameter of A22
  measures "d338" diameter of A23
  measures "d339" diameter of A24
  measures "d340" diameter of A25
  measures "d341" diameter of A26
  measures "d342" distance between parallel lines of L51 L227
  measures "d343" distance between parallel lines of L53 L228
  measures "d344" distance of L227.start L227.end
  measures "d345" distance of L228.start L228.end
  measures "d346" distance edge to line of A26 L230
extrude "押し出し1" add sketch "スケッチ3" against normal blind 1 contours A1 | A2 | A3 | A4 | A5 | L102 L162 L158 | L102 L107 L108 L109 L163 L157 L161 L103 L106 L105 L104 L160 L158 L162 | L102 L109 L108 L107 | L160 L103 L158 | L102 L157 L163 | L104 L105 L106 L103 | L157 L103 L161 | A7 | A10 | A13 | A16 | L164 L165 L181 L180 L179 L229 L245 L221 | L238 L229 L239 L240 L220 L221 | L245 L229 L238 | L238 L239 L229 | L240 L239 L229 L230 L231 L182 L183 L166 L167 L219 L235 L236 L237 L220 | L237 L236 L235 L219 L220 | L195 L194 L242 L186 L185 L184 | L193 L232 L243 L186 L242 | L243 L232 L233 L234 L192 L191 L190 L189 L188 L187 L186 | A19 | A20 | A21 | A22 | A23 | A24 | A25 | A26 | L251 L250 L249 L248 L247 L246 | L246 L267 L259 L272 L271 L251 | L271 L272 L258 | L274 L275 L262 L268 L250 L251 | L261 L275 L274 | L257 L276 L277 L264 L269 L252 | L252 L253 L254 L255 L256 L257 | L263 L277 L276 | L279 L278 L266 | L257 L256 L270 L265 L278 L279
extrude "押し出し2" cut sketch "スケッチ3" against normal blind 1 contours A2 | A3 | A4 | A5
extrude "押し出し3" cut sketch "スケッチ3" against normal blind 1 contours A1
extrude "押し出し4" cut sketch "スケッチ3" against normal up to surface (1 mm away) contours L102 L109 L108 L107 | L104 L105 L106 L103
extrude "押し出し7" cut sketch "スケッチ3" against normal up to surface (1 mm away) contours A7 | A10 | A13 | A16
extrude "押し出し28" cut sketch "スケッチ3" against normal blind 1 contours L102 L162 L158 | L160 L103 L158 | L102 L157 L163 | L157 L103 L161
sketch "スケッチ4" plane through (0, 0, 0) normal (1, 0, 0) x (0, 1, 0)
  circle A0 centre (0, 8.7) radius 10.65 construction
  line L0 (0, 8.7) -> (0, 9.7) construction
  line L1 (0, 8.7) -> (1, 8.7) construction
  circle A1 centre (-13, 8.7) radius 2.25 construction
  circle A2 centre (15.0669, 9.7) radius 4.35 construction
  circle A3 centre (0, 8.7) radius 11.5 construction
  line L2 (-25, -2.8) -> (25, -2.8) construction
  line L3 (-25, -1) -> (25, -1) construction
  line L4 (-25, 0) -> (25, 0) construction
  line L5 (0, -7.4) -> (0, 24.8) projected
  line L6 (-178.8396, 0) -> (401.0377, 0) projected
  point P0 (0, 0)
  point P1 (0, 0)
  dimension "d301" = 1
  dimension "d302" = 1
  dimension "d303" = 21.3
  dimension "d304" = 4.5
  dimension "d306" = 8.7
  dimension "d308" = 23
  dimension "d309" = 50
  dimension "d310" = 1.8
  dimension "d311" = 1
  dimension "d312" = 12.5
  dimension "d313" = 11.5
  dimension "d314" = 0.1
  dimension "d315" = 0.1
  constraints: 10 end point, 5 parallel, 4 centre point, 4 coincident, 3 symmetric about line, 2 midpoint, 1 perpendicular, 1 point on line, 1 tangent, 1 vertical
  measures "d301" distance of L0.start L0.end
  measures "d302" distance of L0.start L1.end
  measures "d303" diameter of A0
  measures "d304" diameter of A1
  measures "d306" diameter of A2
  measures "d308" diameter of A3
  measures "d309" distance of L2.start L2.end
  measures "d310" distance between parallel lines of L2 L3
  measures "d311" distance between parallel lines of L3 L4
  measures "d312" distance from line of L2 A2.centre
  measures "d313" distance from line of L2 A1.centre
extrude "押し出し29" cut sketch "スケッチ3" against normal blind 1 contours A7 | A13 | L164 L165 L181 L180 L179 L229 L245 L221 | L238 L229 L239 L240 L220 L221 | L245 L229 L238 | L240 L239 L229 L230 L231 L182 L183 L166 L167 L219 L235 L236 L237 L220 | L237 L236 L235 L219 L220
extrude "押し出し30" cut sketch "スケッチ3" against normal blind 1 contours A19 | A20 | A23 | A25
extrude "押し出し32" cut sketch "スケッチ3" against normal blind 1 contours L195 L194 L242 L186 L185 L184 | L193 L232 L243 L186 L242 | L243 L232 L233 L234 L192 L191 L190 L189 L188 L187 L186
extrude "押し出し36" add sketch "スケッチ3" against normal blind 1 contours L238 L229 L239 L240 L220 L221 | L245 L229 L238 | L237 L236 L235 L219 L220 | L193 L232 L243 L186 L242
chamfer "面取り6" distance 1 angle 45 3 edges at (-13.5, -24, -0.5) (-15.5392, -29.2108, -0.5) (-12.7108, -32.0392, -0.5)
chamfer "面取り7" distance 2 angle 45 3 edges at (-17, -24, -0.5) (-17, 24, -0.5) (17, 24, -0.5)
chamfer "面取り8" distance 2 angle 45 14 edges at (-17, -14.5, -0.5) (-25.25, -14.5, -0.5) (17, -14.5, -0.5) (25.25, -14.5, -0.5) (3, -30, -0.5) (3, -24, -0.5) (17, -24, -0.5) (-3, 30, -0.5) (-3, 24, -0.5) (13.5, 30, -0.5) (-25.25, 14.5, -0.5) (-17, 14.5, -0.5) (17, 14.5, -0.5) (25.25, 14.5, -0.5)
chamfer "面取り11" distance 1.5 angle 45 4 edges at (-29.25, -8.5, -0.5) (-29.25, 8.5, -0.5) (29.25, 8.5, -0.5) (29.25, -8.5, -0.5)
fillet "フィレット1" radius 0.75 20 edges at (-13.3068, 41.5, -0.5) (13.3068, 41.5, -0.5) (29.25, 20.8653, -0.5) (29.25, 10, -0.5) (27.75, 8.5, -0.5) (17, 8.5, -0.5) (17, -8.5, -0.5) (27.75, -8.5, -0.5) (29.25, -10, -0.5) (29.25, -21.1569, -0.5) (8.9069, -41.5, -0.5) (-8.9069, -41.5, -0.5) (-29.25, -21.1569, -0.5) (-29.25, -10, -0.5) (-27.75, -8.5, -0.5) (-17, -8.5, -0.5) (-17, 8.5, -0.5) (-27.75, 8.5, -0.5) (-29.25, 10, -0.5) (-29.25, 20.8653, -0.5)
fillet "フィレット2" radius 0.75 26 edges at (-19, -14.5, -0.5) (-23.25, -14.5, -0.5) (-25.25, -16.5, -0.5) (-25.25, -19.5, -0.5) (-17, -16.5, -0.5) (-17, -22, -0.5) (-15, -24, -0.5) (-14.5, -24, -0.5) (-13.8644, -24.9312, -0.5) (-15.1748, -28.2796, -0.5) (-16.2463, -28.5037, -0.5) (-7.5, -30, -0.5) (-11.7796, -31.6748, -0.5) (-12.0037, -32.7463, -0.5) (-7.25, -37.5, -0.5) (7.25, -37.5, -0.5) (1, -30, -0.5) (3, -28, -0.5) (3, -26, -0.5) (15, -24, -0.5) (17, -22, -0.5) (17, -16.5, -0.5) (19, -14.5, -0.5) (23.25, -14.5, -0.5) (25.25, -16.5, -0.5) (25.25, -19.5, -0.5)
chamfer "面取り12" distance 2 angle 45 2 edges at (-4.8147, 37.5, -0.5) (4.8147, 37.5, -0.5)
fillet "フィレット3" radius 0.75 31 edges at (10.0926, 30, -0.5) (11.5, 30, -0.5) (13.5, 28, -0.5) (16.1606, 31.2641, -0.5) (25.25, 19.5, -0.5) (25.25, 16.5, -0.5) (23.25, 14.5, -0.5) (19, 14.5, -0.5) (17, 16.5, -0.5) (17, 22, -0.5) (15, 24, -0.5) (13.5, 24, -0.5) (6.0926, 30, -0.5) (5.0634, 31.332, -0.5) (4.8953, 35.5016, -0.5) (2.8147, 37.5, -0.5) (-2.8147, 37.5, -0.5) (-4.8953, 35.5016, -0.5) (-1, 30, -0.5) (-3, 28, -0.5) (-6.1594, 29.9135, -0.5) (-5.0634, 31.332, -0.5) (-3, 26, -0.5) (-16.1606, 31.2641, -0.5) (-15, 24, -0.5) (-17, 16.5, -0.5) (-17, 22, -0.5) (-19, 14.5, -0.5) (-23.25, 14.5, -0.5) (-25.25, 16.5, -0.5) (-25.25, 19.5, -0.5)
extrude "押し出し37" cut sketch "スケッチ3" against normal blind 1 contours L251 L250 L249 L248 L247 L246 | L252 L253 L254 L255 L256 L257
extrude "押し出し39" cut sketch "スケッチ3" against normal blind 1 contours L246 L267 L259 L272 L271 L251 | L271 L272 L258 | L274 L275 L262 L268 L250 L251 | L261 L275 L274 | L257 L276 L277 L264 L269 L252 | L263 L277 L276 | L279 L278 L266 | L257 L256 L270 L265 L278 L279
extrude "押し出し40" add sketch "スケッチ3" against normal blind 1 contours L271 L272 L258 | L261 L275 L274 | L263 L277 L276 | L279 L278 L266
chamfer "面取り14" distance 1 angle 45 4 edges at (-14.5, -13.3971, -0.5) (14.5, -13.3971, -0.5) (14.5, 13.3971, -0.5) (-14.5, 13.3971, -0.5)
fillet "フィレット6" radius 0.75 14 edges at (-13.7246, -14.0286, -0.5) (-14.5, -14.3971, -0.5) (-14.5, -15.3971, -0.5) (-10.5, -20.4081, -0.5) (-7.5, -21.5, -0.5) (7.5, -21.5, -0.5) (10.5, -20.4081, -0.5) (14.5, -15.3971, -0.5) (14.5, -14.3971, -0.5) (13.7246, -14.0286, -0.5) (9.4462, -17.5128, -0.5) (5.3602, -19, -0.5) (-5.3602, -19, -0.5) (-9.4462, -17.5128, -0.5)
mirror "ミラー1" about plane through (0, 0, 0) normal (0, 1, 0) of "フィレット6"
equation "\"d9\" = d8"
equation "\"d11\" = d10"
equation "\"d12\" = d10"
equation "\"d13\" = d10"
equation "\"d15\" = d14"
equation "\"d16\" = d14"
equation "\"d17\" = d10"
